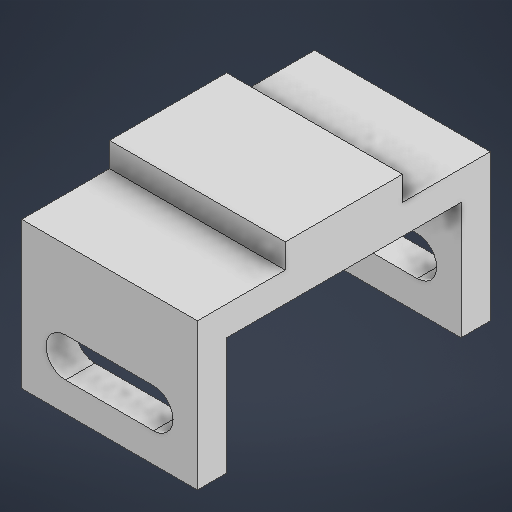
# Autodesk Inventor part: peca1
Saved by Autodesk Inventor 2026 (Build 300175050, 175E)
## iProperties
Created: 2026-04-30
Part Number: peca1
Material: Generic
Document SubType Name: Modeling
Designer: Administrator
Density: 1 g/cm^3
Appearance: Default
Author: Administrator
Autodesk Inventor part; units mm, degrees
ref_plane "YZ Plane" through (0, 0, 0) normal (1, 0, 0) x (0, 1, 0)
ref_plane "XZ Plane" through (0, 0, 0) normal (0, 1, 0) x (-1, 0, 0)
ref_plane "XY Plane" through (0, 0, 0) normal (0, 0, 1) x (1, 0, 0)
sketch "Sketch2" plane through (0, 0, 0) normal (1, 0, 0) x (0, 1, 0)
  line L0 (0, 0) -> (30, 0)
  line L1 (30, 0) -> (30, -18)
  line L2 (30, -18) -> (35, -18)
  line L3 (35, -18) -> (35, -42)
  line L4 (35, -42) -> (30, -42)
  line L5 (30, -42) -> (30, -60)
  line L6 (30, -60) -> (0, -60)
  line L7 (0, -60) -> (0, -54)
  line L8 (0, -54) -> (24, -54)
  line L9 (24, -54) -> (24, -6)
  line L10 (24, -6) -> (0, -6)
  line L11 (0, -6) -> (0, 0)
  dimension "d0" = 60
  dimension "d1" = 6
  dimension "d2" = 6
  dimension "d3" = 18
  dimension "d4" = 24
  dimension "d5" = 30
  dimension "d6" = 24
  dimension "d10" = 35
  constraints: 24 end point, 10 perpendicular, 3 point on line, 1 horizontal
  measures "d0" distance of L6.end L0.start
  measures "d1" distance between parallel lines of L0 L10
  measures "d2" distance between parallel lines of L6 L8
  measures "d3" distance of L0.end L1.end
  measures "d4" distance of L2.end L3.end
  measures "d5" distance of L5.end L6.end
  measures "d6" distance of L7.end L8.end
  measures "d10" horizontal distance of L6.end L3.end
extrude "Extrusion1" add sketch "Sketch2" against normal blind 36
sketch "Sketch3" plane through (0, 0, 0) normal (0, 0, 1) x (1, 0, 0)
  line L0 (0, 0) -> (-36, 0) projected
  line L1 (-27, 0) -> (-27, 10)
  line L2 (-36, 0) -> (-36, 30) projected
  arc A0 (-27, 14) -> (-27, 6) centre (-27, 10) ccw
  line L3 (-27, 10) -> (-9, 10)
  line L4 (-9, 10) -> (-9, 0)
  line L5 (0, 30) -> (0, 0) projected
  arc A1 (-9, 6) -> (-9, 14) centre (-9, 10) ccw
  line L6 (-27, 14) -> (-9, 14)
  line L7 (-27, 6) -> (-9, 6)
  dimension "d11" = 9
  dimension "d12" = 9
  dimension "d13" = 8
  dimension "d14" = 8
  dimension "d15" = 10
  constraints: 10 end point, 4 point on circle, 3 horizontal, 2 centre point, 2 coincident, 2 point on line, 2 tangent, 1 perpendicular, 1 vertical
  measures "d11" distance between parallel lines of L2 L1
  measures "d12" distance between parallel lines of L5 L4
  measures "d13" diameter of A0
  measures "d14" diameter of A1
  measures "d15" distance from line of L0 L1.end
extrude "Extrusion2" cut sketch "Sketch3" against normal through all contours L7 L1 L3 L4 | L4 L3 L1 A0 L6 A1
body "Solid1"
